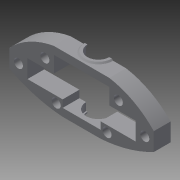
# Autodesk Inventor part: wheel_base
Saved by Autodesk Inventor 2015 (Build 190159000, 159)
## iProperties
Created: 2015-07-19
Part Number: wheel_base
Material: Générique
Document SubType Name: Modeling
Designer: astralien3000
Density: 1 g/cm^3
Appearance: Par défaut
Author: astralien3000
Autodesk Inventor part; units mm, degrees
ref_plane "YZ Plane" through (0, 0, 0) normal (1, 0, 0) x (0, 1, 0)
ref_plane "XZ Plane" through (0, 0, 0) normal (0, 1, 0) x (-1, 0, 0)
ref_plane "XY Plane" through (0, 0, 0) normal (0, 0, 1) x (1, 0, 0)
sketch "Esquisse1" plane through (0, 0, 0) normal (0, 1, 0) x (-1, 0, 0)
  line L0 (0, 5) -> (40, 5)
  line L1 (40, 5) -> (40, -5)
  line L2 (40, -5) -> (0, -5)
  line L3 (0, -5) -> (0, 5)
  line L4 (0, 5) -> (17.5, 5)
  line L5 (17.5, 5) -> (17.5, 19)
  line L6 (17.5, 19) -> (0, 19)
  line L7 (0, 19) -> (0, 5)
  line L8 (0, -5) -> (12.7, -5)
  line L9 (12.7, -5) -> (12.7, -12.2)
  line L10 (12.7, -12.2) -> (0, -12.2)
  line L11 (0, -12.2) -> (0, -5)
  line L12 (17.5, 5) -> (21.5, 5)
  line L13 (21.5, 5) -> (21.5, 7)
  line L14 (21.5, 7) -> (17.5, 7)
  line L15 (17.5, 7) -> (17.5, 5)
  line L16 (12.7, -5) -> (14.7, -5)
  line L17 (14.7, -5) -> (14.7, -7)
  line L18 (14.7, -7) -> (12.7, -7)
  line L19 (12.7, -7) -> (12.7, -5)
  line L20 (40, -5) -> (14.7, -5)
  line L21 (14.7, -5) -> (14.7, -7)
  line L22 (14.7, -7) -> (40, -7)
  line L23 (40, -7) -> (40, -5)
  line L24 (12.7, -12.2) -> (14.7, -12.2)
  line L25 (14.7, -12.2) -> (14.7, -7)
  line L26 (14.7, -7) -> (12.7, -7)
  line L27 (12.7, -7) -> (12.7, -12.2)
  line L28 (40, 5) -> (21.5, 5)
  line L29 (21.5, 5) -> (21.5, 7)
  line L30 (21.5, 7) -> (40, 7)
  line L31 (40, 7) -> (40, 5)
  line L32 (21.5, 7) -> (17.5, 7)
  line L33 (17.5, 7) -> (17.5, 19)
  line L34 (17.5, 19) -> (21.5, 19)
  line L35 (21.5, 19) -> (21.5, 7)
  line L36 (40, -5) -> (42, -5)
  line L37 (42, -5) -> (42, 5)
  line L38 (42, 5) -> (40, 5)
  line L39 (40, 5) -> (40, -5)
  line L40 (0, -12.2) -> (12.7, -12.2)
  line L41 (12.7, -12.2) -> (12.7, -12.7)
  line L42 (12.7, -12.7) -> (0, -12.7)
  line L43 (0, -12.7) -> (0, -12.2)
  line L44 (0, 19) -> (17.5, 19)
  line L45 (17.5, 19) -> (17.5, 19.5)
  line L46 (17.5, 19.5) -> (0, 19.5)
  line L47 (0, 19.5) -> (0, 19)
  line L48 (21.5, 19) -> (17.5, 19)
  line L49 (17.5, 19) -> (17.5, 19.5)
  line L50 (17.5, 19.5) -> (21.5, 19.5)
  line L51 (21.5, 19.5) -> (21.5, 19)
  line L52 (42, 5) -> (40, 5)
  line L53 (40, 5) -> (40, 7)
  line L54 (40, 7) -> (42, 7)
  line L55 (42, 7) -> (42, 5)
  line L56 (42, -5) -> (40, -5)
  line L57 (40, -5) -> (40, -7)
  line L58 (40, -7) -> (42, -7)
  line L59 (42, -7) -> (42, -5)
  line L60 (14.7, -12.2) -> (12.7, -12.2)
  line L61 (12.7, -12.2) -> (12.7, -12.7)
  line L62 (12.7, -12.7) -> (14.7, -12.7)
  line L63 (14.7, -12.7) -> (14.7, -12.2)
  line L64 (0, 19.5) -> (21.5, 19.5)
  line L65 (21.5, 19.5) -> (21.5, 25.5)
  line L66 (21.5, 25.5) -> (0, 25.5)
  line L67 (0, 25.5) -> (0, 19.5)
  line L68 (0, -12.7) -> (14.7, -12.7)
  line L69 (14.7, -12.7) -> (14.7, -18.7)
  line L70 (14.7, -18.7) -> (0, -18.7)
  line L71 (0, -18.7) -> (0, -12.7)
  line L72 (42, -7) -> (56, -7)
  line L73 (56, -7) -> (56, 7)
  line L74 (56, 7) -> (42, 7)
  line L75 (42, 7) -> (42, -7)
  arc A0 (56, 7) -> (21.5, 25.5) centre (10.75, -35.9662) ccw
  arc A1 (21.5, 25.5) -> (0, 25.5) centre (10.75, -35.9662) ccw construction
  arc A2 (0, -18.7) -> (14.7, -18.7) centre (7.35, 85.9876) ccw construction
  arc A3 (14.7, -18.7) -> (56, -7) centre (7.35, 85.9876) ccw
  point P0 (0, 0)
  point P1 (0, 0)
  dimension "d1" = 40
  dimension "d3" = 14
  dimension "d4" = 10
  dimension "d5" = 7.2
  dimension "d6" = 0.5
  dimension "d7" = 0.5
  dimension "d8" = 17.5
  dimension "d9" = 12.7
  dimension "d10" = 2
  dimension "d11" = 2
  dimension "d12" = 2
  dimension "d13" = 4
  dimension "d14" = 2
  dimension "d15" = 6
  dimension "d16" = 6
  dimension "d17" = 14
  constraints: 152 end point, 38 parallel, 19 horizontal, 19 perpendicular, 8 point on circle, 4 centre point, 3 collinear, 1 coincident, 1 midpoint
  measures "d1" distance of L1.end L2.end
  measures "d3" distance of L6.end L0.start
  measures "d4" distance of L2.end L0.start
  measures "d5" distance of L10.end L2.end
  measures "d6" distance of L42.end L10.end
  measures "d7" distance of L46.end L6.end
  measures "d8" distance of L5.end L6.end
  measures "d9" distance of L9.end L10.end
  measures "d10" distance between parallel lines of L36 L58
  measures "d11" distance between parallel lines of L38 L54
  measures "d12" distance between parallel lines of L9 L25
  measures "d13" distance between parallel lines of L33 L35
  measures "d14" distance between parallel lines of L1 L37
  measures "d15" distance between parallel lines of L42 L70
  measures "d16" distance between parallel lines of L46 L66
  measures "d17" distance between parallel lines of L37 L73
extrude "Extrusion1" add sketch "Esquisse1" along normal mid plane 26 contours L67 L66 L65 L50 L46 | L35 L51 L65 A0 L74 L54 L30 | L42 L62 L69 L70 L71 | L55 L74 L73 L72 L59 L37 | L22 L58 L72 A3 L69 L63 L25
mirror "Symétrie1" about plane through (0, 0, 0) normal (1, 0, 0) of "Extrusion1"
sketch "Esquisse4" plane through (-14.7, -13, -18.7) normal (0, 0, -1) x (-1, 0, 0)
  circle A0 centre (-14.7, 13) radius 9.5
  dimension "d25" = 19
  constraints: 1 centre point, 1 coincident
  measures "d25" diameter of A0
extrude "Extrusion4" cut sketch "Esquisse4" against normal through all
sketch "Esquisse5" plane through (0, 13, 0) normal (0, 1, 0) x (1, 0, 0)
  circle A0 centre (19.7, 12) radius 3.5
  circle A1 centre (28.5, -14) radius 3.5
  line L0 (42, 7) -> (56, -7) construction
  line L1 (56, 7) -> (42, -7) construction
  circle A2 centre (49, 0) radius 3.5
  line L2 (21.5, -7) -> (35.5, -7) construction
  line L3 (35.5, -7) -> (35.5, -21) construction
  line L4 (35.5, -21) -> (21.5, -21) construction
  line L5 (21.5, -21) -> (21.5, -7) construction
  line L6 (14.7, 7) -> (24.7, 7) construction
  line L7 (24.7, 7) -> (24.7, 17) construction
  line L8 (24.7, 17) -> (14.7, 17) construction
  line L9 (14.7, 17) -> (14.7, 7) construction
  line L10 (14.7, 17) -> (24.7, 7) construction
  line L11 (24.7, 17) -> (14.7, 7) construction
  line L12 (21.5, -7) -> (35.5, -21) construction
  line L13 (35.5, -7) -> (21.5, -21) construction
  point P0 (0, 0)
  dimension "d28" = 7
  dimension "d29" = 7
  dimension "d36" = 7
  dimension "d37" = 10
  dimension "d38" = 10
  dimension "d39" = 14
  dimension "d40" = 14
  dimension "d41" = 14
  dimension "d60" = 28.5
  constraints: 28 end point, 4 midpoint, 4 parallel, 3 centre point, 3 perpendicular, 2 horizontal, 1 coincident
  measures "d28" diameter of A0
  measures "d29" diameter of A1
  measures "d36" diameter of A2
  measures "d37" distance of L7.end L8.end
  measures "d38" distance of L6.end L7.end
  measures "d39" distance of L3.end L4.end
  measures "d40" distance of L2.end L3.end
  measures "d41" distance of L1.start L0.end
  measures "d60" horizontal distance of point (0, 0) A1.centre
extrude "Extrusion5" cut sketch "Esquisse5" against normal through all
mirror "Symétrie3" about plane through (0, 0, 0) normal (1, 0, 0) of "Extrusion5"
sketch "Esquisse7" plane through (-21.5, -13, 25.5) normal (0, 0, 1) x (1, 0, 0)
  circle A0 centre (21.5, 13) radius 9.5 projected
  circle A1 centre (21.5, 13) radius 8.5
  circle A2 centre (21.5, 13) radius 11.5
  dimension "d44" = 1
  dimension "d45" = 2
  constraints: 2 centre point, 2 coincident
  measures "d44" radial gap between concentric circles of A0 A1
  measures "d45" radial gap between concentric circles of A2 A0
extrude "Extrusion7" add sketch "Esquisse7" along normal blind 1 contours A0 | A2
chamfer "Chanfrein1" distance 1 angle 45 1 edges at (-11.5, 0, 26.5)
sketch "Esquisse8" plane through (-14.7, -13, -18.7) normal (0, 0, -1) x (-1, 0, 0)
  circle A0 centre (-14.7, 13) radius 9.5 projected
  circle A1 centre (-14.7, 13) radius 11.5
  circle A2 centre (-14.7, 13) radius 8.5
  dimension "d51" = 1
  dimension "d52" = 2
  constraints: 2 centre point, 2 coincident
  measures "d51" radial gap between concentric circles of A0 A2
  measures "d52" radial gap between concentric circles of A1 A0
extrude "Extrusion8" add sketch "Esquisse8" along normal blind 1 contours A0 | A1
chamfer "Chanfrein2" distance 1 angle 45 1 edges at (11.5, 0, -19.7)
sketch "Esquisse9" plane through (0, 0, 26.5) normal (0, 0, 1) x (1, 0, 0)
  circle A0 centre (0, 0) radius 8.5 projected
  line L0 (-56, 13) -> (56, 13)
  line L1 (56, 13) -> (56, 0)
  line L2 (56, 0) -> (-56, 0)
  line L3 (-56, 0) -> (-56, 13)
  line L4 (-56, -13) -> (-56, 13) projected
  line L5 (56, -13) -> (56, 13) projected
  line L6 (-21.5, 13) -> (21.5, 13) projected
  constraints: 8 end point, 3 collinear, 2 parallel, 1 horizontal, 1 midpoint, 1 perpendicular
extrude "Extrusion9" cut sketch "Esquisse9" against normal through all contours L2 A0 | A0 L2 L3 L0 L1 picked at (2.1208, 1.8788)
